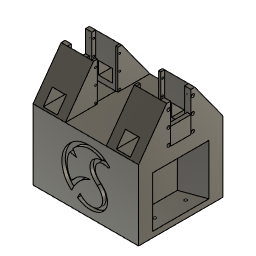
dual_motor_plate v1 (Autodesk Fusion 360 design; units mm, degrees)
Autodesk Fusion 360 part; units mm, degrees
sketch "스케치2" plane through (0, 0, 0) normal (0, 0, 1) x (1, 0, 0)
  line L0 (0, 0) -> (150, 0)
  line L1 (150, 0) -> (150, 120)
  line L2 (150, 120) -> (0, 120)
  line L3 (0, 120) -> (0, 0)
  circle A0 centre (15, 82) radius 2
  circle A1 centre (15, 38) radius 2
  circle A2 centre (135, 82) radius 2
  circle A3 centre (135, 38) radius 2
  line L4 (0, 120) -> (0, 100) construction
  line L5 (0, 0) -> (0, 20) construction
  line L6 (0, 100) -> (35, 100) construction
  line L7 (0, 20) -> (35, 20) construction
  line L8 (32.8892, 88.0293) -> (32.8892, 31.9707) construction
  line L9 (150, 120) -> (150, 100) construction
  line L10 (150, 120) -> (150, 100) construction
  line L11 (32.8892, 88.0293) -> (32.8892, 31.9707)
  line L12 (117.1108, 88.0293) -> (117.1108, 31.9707)
  line L13 (32.8892, 88.0293) -> (0, 100)
  line L14 (32.8892, 31.9707) -> (0, 20)
  line L15 (117.1108, 88.0293) -> (150, 100)
  line L16 (117.1108, 31.9707) -> (150, 20)
  dimension "d15" = 150
  dimension "d16" = 120
  dimension "d19" = 120
  dimension "d20" = 44
  dimension "d21" = 4
  dimension "d22" = 4
  dimension "d23" = 4
  dimension "d24" = 4
  dimension "d98" = 20
  dimension "d99" = 20
  dimension "d100" = 35
  dimension "d102" = 35
  dimension "d105" = 35
  constraint horizontal L0
  constraint vertical L1
  constraint horizontal L2
  constraint vertical L3
  constraint coincident L0.start L3.end
  constraint perpendicular L2 L4
  constraint perpendicular L0 L5
  constraint horizontal L6
  constraint horizontal L7
  constraint coincident L1 L9.end
  constraint parallel L14 L15
  constraint coincident L1 L16.end
  constraint parallel L13 L16
  measures "d15" distance of L0.start L0.end
  measures "d16" distance of L0.start L2.end
  measures "d19" distance of A0.centre A2.centre
  measures "d20" distance of A2.centre A3.centre
  measures "d21" diameter of A0
  measures "d22" diameter of A1
  measures "d23" diameter of A2
  measures "d24" diameter of A3
  measures "d98" distance of L2.end L4.end
  measures "d99" distance of L0.start L5.end
  measures "d100" distance of L4.end L8.start
  measures "d102" distance of L5.end L8.end
  measures "d105" distance of L9.end L12.start
sketch "스케치3" plane through (0, 0, 100) normal (0, 0, 1) x (-1, 0, 0)
  circle A0 centre (-135, -82) radius 2
  circle A1 centre (-15, -82) radius 2
  circle A2 centre (-15, -38) radius 2
  circle A3 centre (-135, -38) radius 2
  line L0 (0, -120) -> (0, 0)
  line L1 (0, 0) -> (-150, 0)
  line L2 (-150, 0) -> (-150, -120)
  line L3 (-150, -120) -> (0, -120)
  line L4 (0, -60) -> (-150, -60) construction
  line L5 (0, -60) -> (-5.5, -60) construction
  line L6 (-5.5, -60) -> (-46.5, -60) construction
  line L7 (-46.5, -60) -> (-103.5, -60) construction
  line L8 (-103.5, -60) -> (-144.5, -60) construction
  line L9 (-144.5, -60) -> (-150, -60) construction
  line L10 (-5.5, -60) -> (-26, -60) construction
  line L11 (-26, -60) -> (-9, -60) construction
  line L12 (-9, -60) -> (-43, -60) construction
  line L13 (-144.5, -60) -> (-124, -60) construction
  line L14 (-124, -60) -> (-141, -60) construction
  line L15 (-141, -60) -> (-107, -60) construction
  line L16 (-46.5, -60) -> (-26, -60) construction
  line L17 (-9, -60) -> (-43, -60) construction
  line L18 (-43, -60) -> (-43, -80) construction
  line L19 (-43, -80) -> (-9, -80) construction
  line L20 (-9, -80) -> (-9, -60) construction
  line L21 (-43, -80) -> (-9, -80)
  line L22 (-9, -80) -> (-9, -40)
  line L23 (-9, -40) -> (-43, -40)
  line L24 (-43, -40) -> (-43, -80)
  line L25 (-107, -60) -> (-141, -60) construction
  line L26 (-141, -60) -> (-141, -40) construction
  line L27 (-141, -40) -> (-107, -40)
  line L28 (-107, -40) -> (-107, -60) construction
  line L29 (-107, -40) -> (-141, -40) construction
  line L30 (-141, -40) -> (-141, -80)
  line L31 (-141, -80) -> (-107, -80)
  line L32 (-107, -80) -> (-107, -40)
  dimension "d27" = 5.5
  dimension "d28" = 41
  dimension "d29" = 57
  dimension "d30" = 41
  dimension "d31" = 5.5
  dimension "d34" = 34
  dimension "d37" = 34
  dimension "d38" = 34
  dimension "d39" = 20
  dimension "d40" = 34
  dimension "d41" = 40
  dimension "d42" = 34
  dimension "d43" = 20
  dimension "d44" = 34
  dimension "d45" = 40
  constraint midpoint L0 L4.start
  constraint midpoint L2 L4.end
  constraint perpendicular L0 L5
  constraint perpendicular L0 L6
  constraint parallel L4 L7
  constraint perpendicular L0 L8
  constraint perpendicular L2 L9
  constraint parallel L4 L10
  constraint parallel L10 L11
  constraint parallel L6 L12
  constraint midpoint L8 L13.end
  constraint parallel L8 L14
  constraint parallel L8 L15
  constraint parallel L12 L16
  constraint horizontal L17
  constraint vertical L18
  constraint horizontal L19
  constraint vertical L20
  constraint horizontal L21
  constraint vertical L22
  constraint horizontal L23
  constraint vertical L24
  constraint horizontal L25
  constraint vertical L26
  constraint horizontal L27
  constraint vertical L28
  constraint horizontal L29
  constraint vertical L30
  constraint horizontal L31
  constraint vertical L32
  measures "d27" distance of L4.start L5.end
  measures "d28" distance of L5.end L6.end
  measures "d29" distance of L6.end L7.end
  measures "d30" distance of L7.end L8.end
  measures "d31" distance of L8.end L4.end
  measures "d34" distance of L11.end L12.end
  measures "d37" distance of L14.end L15.end
  measures "d38" distance of L11.end L12.end
  measures "d39" distance of L11.end L19.end
  measures "d40" distance of L18.end L19.end
  measures "d41" distance of L18.end L23.end
  measures "d42" distance of L15.end L14.end
  measures "d43" distance of L15.end L27.end
  measures "d44" distance of L27.end L26.end
  measures "d45" distance of L27.end L31.end
extrude "돌출3" add sketch "스케치2" along normal blind 100 contours L0 L1 L2 L3 L11 L12 L13 L14 L15 L16 | L3 L11 L13 L14 | L1 L12 L15 L16 | A0 | A1 | A2 | A3 makes body 1
extrude "돌출4" cut sketch "스케치3" against normal blind 5.6 contours L27 L30 L31 L32 | L21 L22 L23 L24 bodies 1
sketch "스케치4" plane through (150, 0, 0) normal (1, 0, 0) x (0, 1, 0)
  line L0 (0, 0) -> (120, 0)
  line L1 (120, 0) -> (120, 100)
  line L2 (120, 100) -> (0, 100)
  line L3 (0, 100) -> (0, 0)
  line L4 (40, 100) -> (80, 100)
  line L5 (40, 100) -> (40, 155.5) construction
  line L6 (80, 100) -> (80, 155.5)
  line L7 (40, 100) -> (45.5, 100)
  line L8 (80, 100) -> (74.5, 100)
  line L9 (45.5, 100) -> (40, 100)
  line L10 (40, 100) -> (40, 155.5)
  line L11 (40, 155.5) -> (45.5, 155.5)
  line L12 (45.5, 155.5) -> (45.5, 100)
  line L13 (74.5, 100) -> (80, 100)
  line L14 (80, 100) -> (80, 155.5) construction
  line L15 (80, 155.5) -> (74.5, 155.5)
  line L16 (74.5, 155.5) -> (74.5, 100)
  line L17 (40, 155.5) -> (0, 100)
  line L18 (80, 155.5) -> (120, 100)
  line L19 (42.75, 155.5) -> (42.75, 146.5) construction
  line L20 (42.75, 146.5) -> (42.75, 124.5) construction
  line L21 (42.75, 124.5) -> (42.75, 102.5) construction
  circle A0 centre (42.75, 146.5) radius 1.25
  circle A1 centre (42.75, 124.5) radius 1.25
  circle A2 centre (42.75, 102.5) radius 1.25
  line L22 (77.25, 155.5) -> (77.25, 146.5) construction
  line L23 (77.25, 146.5) -> (77.25, 124.5) construction
  line L24 (77.25, 124.5) -> (77.25, 102.5) construction
  circle A3 centre (77.25, 146.5) radius 1.25
  circle A4 centre (77.25, 124.5) radius 1.25
  circle A5 centre (77.25, 102.5) radius 1.25
  circle A6 centre (42.75, 146.5) radius 2.25
  circle A7 centre (42.75, 124.5) radius 2.25
  circle A8 centre (42.75, 102.5) radius 2.25
  circle A9 centre (77.25, 102.5) radius 2.25
  circle A10 centre (77.25, 124.5) radius 2.25
  circle A11 centre (77.25, 146.5) radius 2.25
  line L25 (45.5, 124.5) -> (74.5, 124.5)
  line L26 (74.5, 124.5) -> (74.5, 100)
  line L27 (74.5, 100) -> (45.5, 100)
  line L28 (45.5, 100) -> (45.5, 124.5)
  dimension "d50" = 55.5
  dimension "d51" = 55.5
  dimension "d52" = 5.5
  dimension "d53" = 5.5
  dimension "d54" = 9
  dimension "d55" = 22
  dimension "d56" = 22
  dimension "d57" = 2.5
  dimension "d58" = 2.5
  dimension "d59" = 2.5
  dimension "d60" = 9
  dimension "d61" = 22
  dimension "d62" = 22
  dimension "d63" = 2.5
  dimension "d64" = 2.5
  dimension "d65" = 2.5
  dimension "d74" = 4.5
  dimension "d75" = 4.5
  dimension "d76" = 4.5
  dimension "d77" = 4.5
  dimension "d78" = 4.5
  dimension "d79" = 4.5
  constraint coincident L2 L4.start
  constraint coincident L2 L4.end
  constraint perpendicular L3 L4
  constraint perpendicular L4 L5
  constraint perpendicular L4 L6
  constraint perpendicular L5 L7
  constraint perpendicular L6 L8
  constraint horizontal L9
  constraint vertical L10
  constraint horizontal L11
  constraint vertical L12
  constraint horizontal L13
  constraint vertical L14
  constraint horizontal L15
  constraint vertical L16
  constraint coincident L2.end L3.start
  constraint coincident L1.end L2.start
  constraint midpoint L11 L19.start
  constraint perpendicular L11 L19
  constraint parallel L10 L20
  constraint parallel L12 L21
  constraint coincident L19.end L20.start
  constraint coincident L20.end L21.start
  constraint coincident L21.end A2.centre
  constraint midpoint L15 L22.start
  constraint perpendicular L15 L22
  constraint parallel L22 L23
  constraint parallel L23 L24
  constraint coincident L22.end L23.start
  constraint coincident L23.end L24.start
  constraint coincident L24.end A5.centre
  constraint concentric A0 A6
  constraint concentric A1 A7
  constraint concentric A2 A8
  constraint concentric A5 A9
  constraint concentric A3 A11
  constraint horizontal L25
  constraint vertical L26
  constraint horizontal L27
  constraint vertical L28
  constraint coincident L12 L25.start
  measures "d50" distance of L4.start L5.end
  measures "d51" distance of L4.end L6.end
  measures "d52" distance of L4.start L7.end
  measures "d53" distance of L4.end L8.end
  measures "d54" distance of L19.start L19.end
  measures "d55" distance of L19.end L20.end
  measures "d56" distance of L20.end L21.end
  measures "d57" diameter of A0
  measures "d58" diameter of A1
  measures "d59" diameter of A2
  measures "d60" distance of L22.start L22.end
  measures "d61" distance of L22.end L23.end
  measures "d62" distance of L23.end L24.end
  measures "d63" diameter of A3
  measures "d64" diameter of A4
  measures "d65" diameter of A5
  measures "d74" diameter of A6
  measures "d75" diameter of A7
  measures "d76" diameter of A8
  measures "d77" diameter of A9
  measures "d78" diameter of A10
  measures "d79" diameter of A11
extrude "돌출5" add sketch "스케치4" along normal blind 3 separate body contours L2 L10 L17 | L2 L6 L18 | L2 L4 L7 L9 L10 L11 L12 L28 | L2 L4 L6 L8 L13 L15 L16 L26 | A6 | A7 | A8 | A9 | A10 | A11 makes body 2 at (150, 27.7492, 109) makes body 3 at (150, 92.2508, 109)
combine "결합1" operation add target body 2 tool bodies 3 makes body 4 at (150, 92.2508, 109)
move_body "이동1" bodies 2 4 to x (1, 0, 0) y (0, 1, 0) z (0, 0, 1) at (-9, 0, 0)
copy_body "CopyPasteBodies1" bodies 2 4 makes body 5 makes body 6
move_body "이동2" bodies 5 6 to x (1, 0, 0) y (0, 1, 0) z (0, 0, 1) at (-37, 0, 0)
copy_body "CopyPasteBodies2" bodies 2 6 5 4 makes body 7 makes body 8 makes body 9 makes body 10
move_body "이동3" bodies 7 8 10 9 to x (1, 0, 0) y (0, 1, 0) z (0, 0, 1) at (-98, 0, 0)
extrude "돌출7" add 1 faces at (144, 27.7492, 109) along direction (1, 0, 0) up to surface (6 mm away) on bodies 2 bodies 2 4 5 6 7 8 9 10 1
extrude "돌출8" add 1 faces at (144, 92.2508, 109) along direction (1, 0, 0) blind 6 on bodies 4 bodies 4 5 6 7 8 9 10 2
extrude "돌출9" cut sketch "스케치4" against normal blind 6 contours A0 | A1 | A2 | A3 | A4 | A5 | A6 | A7 | A8 | A9 | A10 | A11 bodies 4
extrude "돌출10" add sketch "스케치4" along normal blind 6 separate body contours L2 L10 L17 | L2 L6 L18 | L2 L4 L7 L9 L10 L11 L12 L28 | L2 L4 L6 L8 L13 L15 L16 L26 makes body 11 at (150, 27.1485, 109) makes body 12 at (150, 92.8515, 109)
move_body "이동4" bodies 11 12 to x (1, 0, 0) y (0, 1, 0) z (0, 0, 1) at (-150, 0, 0)
combine "결합2" operation add target body 12 tool bodies 8 11 9 makes body 13 at (9, 27.7492, 109)
extrude "돌출11" add sketch "스케치4" against normal blind 43 contours L2 L10 L17 | L2 L6 L18 bodies 4 5 6
extrude "돌출12" add sketch "스케치4" along normal blind 34 separate body contours L2 L10 L17 | L2 L6 L18 makes body 14 at (161.3333, 93.3333, 137) makes body 15 at (161.3333, 26.6667, 137)
move_body "이동5" bodies 15 14 to x (1, 0, 0) y (0, 1, 0) z (0, 0, 1) at (-141, 0, 0)
extrude "돌출13" add sketch "스케치4" against normal blind 5.4 separate body contours L2 L4 L12 L16 L25 L26 L27 L28 makes body 16
copy_body "CopyPasteBodies3" bodies 16 makes body 17
move_body "이동6" bodies 17 to x (1, 0, 0) y (0, 1, 0) z (0, 0, 1) at (-144.6, 0, 0)
sketch "스케치5" plane through (0, 0, 0) normal (0, -1, 0) x (1, 0, 0)
  line L0 (0, 0) -> (150, 0)
  line L1 (150, 0) -> (150, 100)
  line L2 (150, 100) -> (104, 100)
  line L3 (104, 100) -> (0, 100)
  line L4 (0, 100) -> (0, 0)
  line L5 (127, 100) -> (117, 100)
  line L6 (117, 120) -> (137, 120)
  line L7 (137, 120) -> (137, 102)
  line L8 (137, 102) -> (117, 102)
  line L9 (117, 102) -> (117, 120)
  line L10 (13, 102) -> (33, 102)
  line L11 (33, 102) -> (33, 120)
  line L12 (33, 120) -> (13, 120)
  line L13 (13, 120) -> (13, 102)
  dimension "d90" = 20
  dimension "d92" = 20
  dimension "d94" = 20
  dimension "d95" = 18
  constraint midpoint L2 L5.start
  constraint coincident L2 L5.end
  constraint perpendicular L1 L5
  constraint horizontal L6
  constraint vertical L7
  constraint horizontal L8
  constraint vertical L9
  constraint horizontal L10
  constraint vertical L11
  constraint horizontal L12
  constraint vertical L13
  measures "d90" distance of L5.end L6.start
  measures "d92" distance of L6.start L6.end
  measures "d94" distance of L10.start L10.end
  measures "d95" distance of L10.start L12.end
combine "결합3" operation add target body 15 tool bodies 14 13 12 10 7 4
extrude "돌출14" cut sketch "스케치5" against normal blind 120 contours L6 L7 L8 L9 | L10 L11 L12 L13 bodies 15
sketch "스케치6" plane through (0, 120, 0) normal (0, 1, 0) x (-1, 0, 0)
  line L0 (-150, 0) -> (0, 0)
  line L1 (0, 0) -> (0, 100)
  line L2 (0, 100) -> (-46, 100)
  line L3 (-46, 100) -> (-104, 100)
  line L4 (-104, 100) -> (-150, 100)
  line L5 (-150, 100) -> (-150, 0)
  line L6 (-110, 84) -> (-40, 84)
  line L7 (-40, 84) -> (-40, 16)
  line L8 (-40, 16) -> (-110, 16)
  line L9 (-110, 16) -> (-110, 84)
  line L10 (-75, 80.8) -> (-102.5, 80.8) construction
  line L11 (-102.5, 80.8) -> (-47.5, 80.8) construction
  line L12 (-47.5, 80.8) -> (-47.5, 19.2) construction
  line L13 (-47.5, 19.2) -> (-102.5, 19.2) construction
  line L14 (-102.5, 19.2) -> (-102.5, 80.8) construction
  circle A0 centre (-102.5, 80.8) radius 1.5
  circle A1 centre (-47.5, 80.8) radius 1.5
  circle A2 centre (-102.5, 19.2) radius 1.5
  circle A3 centre (-47.5, 19.2) radius 1.5
  dimension "d110" = 70
  dimension "d111" = 68
  dimension "d116" = 55
  dimension "d117" = 61.6
  dimension "d118" = 3
  dimension "d119" = 3
  dimension "d120" = 3
  dimension "d121" = 3
  constraint horizontal L6
  constraint vertical L7
  constraint horizontal L8
  constraint vertical L9
  constraint horizontal L11
  constraint vertical L12
  constraint horizontal L13
  constraint vertical L14
  constraint coincident L10.end L11.start
  constraint coincident L11.end L12.start
  constraint coincident L13.end L14.start
  constraint coincident L12.end L13.start
  measures "d110" distance of L6.start L6.end
  measures "d111" distance of L6.start L8.end
  measures "d116" distance of L10.end L11.end
  measures "d117" distance of L10.end L13.end
  measures "d118" diameter of A0
  measures "d119" diameter of A1
  measures "d120" diameter of A2
  measures "d121" diameter of A3
extrude "돌출15" cut sketch "스케치6" against normal blind 5 contours L6 L7 L8 L9 | A0 | A1 | A2 | A3 bodies 15
extrude "돌출16" cut sketch "스케치6" against normal blind 10 contours A0 | A1 | A2 | A3 bodies 15
extrude "돌출17" cut sketch "스케치2" along normal blind 80 contours L3 L11 L13 L14 | L1 L12 L15 L16 | A0 | A1 | A2 | A3 bodies 15
extrude "돌출18" add sketch "스케치2" along normal blind 8 contours L3 L11 L13 L14 | L1 L12 L15 L16 bodies 15
sketch "스케치7" plane through (0, 0, 0) normal (0, -1, 0) x (1, 0, 0)
  line L0 (0, 0) -> (150, 0)
  line L1 (150, 0) -> (150, 100)
  line L2 (150, 100) -> (104, 100)
  line L3 (104, 100) -> (46, 100)
  line L4 (46, 100) -> (0, 100)
  line L5 (0, 100) -> (0, 0)
sketch "스케치8" plane through (75, 0, 50) normal (0, -1, 0) x (1, 0, 0)
  spline S0 degree 5 poles (-20.1512, -28.9535) (-20.3666, -28.7887) (-20.8036, -28.4443) (-21.4782, -27.8837) (-22.4158, -27.0479) (-23.6508, -25.8441) (-24.9472, -24.4441) (-26.2998, -22.7858) (-27.6927, -20.8074) (-29.0947, -18.466) (-30.4521, -15.7602) (-31.6969, -12.7202) (-32.755, -9.398) (-33.5542, -5.8575) (-34.0317, -2.165) (-34.1436, 1.621) (-33.8627, 5.4488) (-33.1759, 9.2713) (-32.0819, 13.0444) (-30.5889, 16.7249) (-28.7125, 20.2689) (-26.474, 23.6297) (-23.8981, 26.7595) (-21.0116, 29.6118) (-17.8418, 32.143) (-14.4143, 34.3146) (-10.7522, 36.0953) (-6.8741, 37.4635) (-2.7941, 38.4064) (1.4776, 38.9177) (5.9341, 38.9955) (9.6436, 38.7117) (12.5061, 38.305) (14.4501, 37.9479) (15.4309, 37.7479) knots 0 0 0 0 0 0 0.033333 0.066667 0.1 0.133333 0.166667 0.2 0.233333 0.266667 0.3 0.333333 0.366667 0.4 0.433333 0.466667 0.5 0.533333 0.566667 0.6 0.633333 0.666667 0.7 0.733333 0.766667 0.8 0.833333 0.866667 0.9 0.933333 0.966667 1 1 1 1 1 1
  spline S1 degree 5 poles (15.4309, 37.7479) (15.6205, 37.7339) (16.0093, 37.6921) (16.6216, 37.5882) (17.4968, 37.3668) (18.6893, 36.9498) (19.977, 36.3929) (21.3504, 35.7016) (22.7884, 34.8915) (24.2597, 33.9875) (25.7275, 33.0192) (27.1535, 32.018) (28.502, 31.0132) (29.7439, 30.0294) (30.8625, 29.0822) (31.8507, 28.1797) (32.5363, 27.496) (32.9922, 27.0049) (33.2703, 26.687) (33.4029, 26.5305) knots 0 0 0 0 0 0 0.066667 0.133333 0.2 0.266667 0.333333 0.4 0.466667 0.533333 0.6 0.666667 0.733333 0.8 0.866667 0.933333 1 1 1 1 1 1
  spline S2 degree 5 poles (33.4029, 26.5305) (33.4205, 26.4745) (33.4487, 26.3561) (33.4707, 26.1597) (33.4592, 25.8606) (33.3718, 25.4401) (33.1937, 25.0294) (32.8993, 24.714) (32.4701, 24.5642) (31.9107, 24.5893) (31.2465, 24.7436) (30.5109, 24.9601) (29.7369, 25.1747) (28.9454, 25.3561) (28.1471, 25.498) (27.3449, 25.608) (26.5357, 25.6985) (25.7123, 25.7757) (24.866, 25.8322) (23.9882, 25.8516) (23.0728, 25.8122) (22.118, 25.6905) (21.1289, 25.4655) (20.119, 25.1217) (19.108, 24.6488) (18.1191, 24.0417) (17.1775, 23.3004) (16.3073, 22.4291) (15.5299, 21.4368) (14.8611, 20.337) (14.3118, 19.1464) (13.8885, 17.8841) (13.5945, 16.5704) (13.4306, 15.2255) (13.3959, 13.8686) (13.4882, 12.5166) (13.7055, 11.1831) (14.046, 9.8779) (14.5079, 8.608) (15.0898, 7.3779) (15.7905, 6.1901) (16.4455, 5.2747) (16.9895, 4.6078) (17.3757, 4.172) (17.5747, 3.9563) knots 0 0 0 0 0 0 0.025 0.05 0.075 0.1 0.125 0.15 0.175 0.2 0.225 0.25 0.275 0.3 0.325 0.35 0.375 0.4 0.425 0.45 0.475 0.5 0.525 0.55 0.575 0.6 0.625 0.65 0.675 0.7 0.725 0.75 0.775 0.8 0.825 0.85 0.875 0.9 0.925 0.95 0.975 1 1 1 1 1 1
  spline S3 degree 5 poles (17.5747, 3.9563) (17.6741, 3.8277) (17.8885, 3.5636) (18.2573, 3.1465) (18.8433, 2.5486) (19.7281, 1.7294) (20.7502, 0.8335) (21.8784, -0.1497) (23.0699, -1.2323) (24.2769, -2.4237) (25.4522, -3.7271) (26.5556, -5.1338) (27.5578, -6.6232) (28.4379, -8.1696) (29.1833, -9.7476) (29.788, -11.3375) (30.2521, -12.9326) (30.58, -14.54) (30.7767, -16.1736) (30.8449, -17.8481) (30.7817, -19.5736) (30.5749, -21.3484) (30.2051, -23.1596) (29.6508, -24.9867) (28.8931, -26.8039) (27.92, -28.5832) (26.7315, -30.2974) (25.3412, -31.9215) (23.7711, -33.433) (22.0488, -34.8119) (20.2036, -36.0406) (18.2635, -37.105) (16.2506, -37.9935) (14.1805, -38.6983) (12.0651, -39.2153) (9.9145, -39.5441) (7.7396, -39.689) (5.554, -39.6589) (3.3762, -39.4679) (1.2312, -39.1351) (-0.8537, -38.682) (-2.8501, -38.131) (-4.7313, -37.5035) (-6.4747, -36.8178) (-8.0644, -36.087) (-9.4914, -35.319) (-10.4995, -34.678) (-11.1799, -34.1828) (-11.6, -33.8464) (-11.8016, -33.6766) knots 0 0 0 0 0 0 0.022222 0.044444 0.066667 0.088889 0.111111 0.133333 0.155556 0.177778 0.2 0.222222 0.244444 0.266667 0.288889 0.311111 0.333333 0.355556 0.377778 0.4 0.422222 0.444444 0.466667 0.488889 0.511111 0.533333 0.555556 0.577778 0.6 0.622222 0.644444 0.666667 0.688889 0.711111 0.733333 0.755556 0.777778 0.8 0.822222 0.844444 0.866667 0.888889 0.911111 0.933333 0.955556 0.977778 1 1 1 1 1 1
  line L0 (-11.8016, -33.6766) -> (-8.1599, -26.9758)
  spline S4 degree 5 poles (-8.1599, -26.9758) (-8.0677, -27.0973) (-7.8739, -27.3434) (-7.5554, -27.722) (-7.0748, -28.246) (-6.3818, -28.9313) (-5.5992, -29.6427) (-4.734, -30.3707) (-3.7948, -31.1018) (-2.7893, -31.8188) (-1.7215, -32.5026) (-0.5877, -33.1329) (0.6216, -33.6896) (1.9161, -34.1547) (3.3001, -34.5144) (4.7673, -34.7606) (6.2945, -34.893) (7.8461, -34.9174) (9.3824, -34.8426) (10.8664, -34.6771) (12.2709, -34.4266) (13.5873, -34.0905) (14.8248, -33.6618) (16.0009, -33.1299) (17.134, -32.4828) (18.2361, -31.7094) (19.3035, -30.8019) (20.3208, -29.7565) (21.2642, -28.5734) (22.1063, -27.2572) (22.8195, -25.8173) (23.3806, -24.2686) (23.7709, -22.6299) (23.9755, -20.9221) (23.9832, -19.1666) (23.7853, -17.3837) (23.376, -15.5908) (22.7516, -13.8008) (21.9099, -12.023) (20.8503, -10.2633) (19.5728, -8.5252) (18.377, -7.1534) (17.3826, -6.1353) (16.6763, -5.4614) (16.3124, -5.1256) knots 0 0 0 0 0 0 0.025 0.05 0.075 0.1 0.125 0.15 0.175 0.2 0.225 0.25 0.275 0.3 0.325 0.35 0.375 0.4 0.425 0.45 0.475 0.5 0.525 0.55 0.575 0.6 0.625 0.65 0.675 0.7 0.725 0.75 0.775 0.8 0.825 0.85 0.875 0.9 0.925 0.95 0.975 1 1 1 1 1 1
  spline S5 degree 5 poles (16.3124, -5.1256) (16.147, -4.988) (15.8142, -4.7057) (15.3085, -4.2605) (14.6212, -3.6235) (13.7414, -2.755) (12.845, -1.8155) (11.9396, -0.8076) (11.0387, 0.2637) (10.1608, 1.3912) (9.3268, 2.5672) (8.5577, 3.7842) (7.8719, 5.0362) (7.2828, 6.3204) (6.7974, 7.6369) (6.4186, 8.9868) (6.1465, 10.3699) (5.9808, 11.7828) (5.9219, 13.217) (5.9726, 14.6569) (6.1365, 16.0837) (6.4174, 17.4772) (6.818, 18.8192) (7.3389, 20.0954) (7.9776, 21.2988) (8.7291, 22.4268) (9.5861, 23.4796) (10.5399, 24.4578) (11.5799, 25.3608) (12.6951, 26.1847) (13.8739, 26.9235) (15.1056, 27.5705) (16.3802, 28.1188) (17.69, 28.563) (19.0298, 28.8998) (20.3962, 29.1277) (21.5094, 29.2224) (22.3552, 29.2444) (22.9239, 29.2372) (23.2095, 29.2281) knots 0 0 0 0 0 0 0.028571 0.057143 0.085714 0.114286 0.142857 0.171429 0.2 0.228571 0.257143 0.285714 0.314286 0.342857 0.371429 0.4 0.428571 0.457143 0.485714 0.514286 0.542857 0.571429 0.6 0.628571 0.657143 0.685714 0.714286 0.742857 0.771429 0.8 0.828571 0.857143 0.885714 0.914286 0.942857 0.971429 1 1 1 1 1 1
  spline S6 degree 5 poles (23.2095, 29.2281) (23.1228, 29.3204) (22.934, 29.5059) (22.6042, 29.7871) (22.0713, 30.1676) (21.2528, 30.6514) (20.292, 31.1391) (19.2109, 31.6224) (18.0391, 32.0901) (16.8085, 32.5316) (15.5489, 32.9383) (14.2816, 33.307) (13.0184, 33.6389) (11.7617, 33.9358) (10.5047, 34.1974) (9.2313, 34.4181) (7.9163, 34.5845) (6.5307, 34.6781) (5.048, 34.6792) (3.4492, 34.5695) (1.7287, 34.3358) (-0.1008, 33.9727) (-2.0137, 33.4806) (-3.9751, 32.8642) (-5.9455, 32.1314) (-7.8849, 31.2913) (-9.7564, 30.3533) (-11.5315, 29.3253) (-13.191, 28.2133) (-14.7227, 27.0216) (-16.1201, 25.7531) (-17.1283, 24.6784) (-17.8226, 23.839) (-18.2581, 23.2646) (-18.4689, 22.9737) knots 0 0 0 0 0 0 0.033333 0.066667 0.1 0.133333 0.166667 0.2 0.233333 0.266667 0.3 0.333333 0.366667 0.4 0.433333 0.466667 0.5 0.533333 0.566667 0.6 0.633333 0.666667 0.7 0.733333 0.766667 0.8 0.833333 0.866667 0.9 0.933333 0.966667 1 1 1 1 1 1
  line L1 (-18.4689, 22.9737) -> (-13.116, 14.972)
  line L2 (-13.116, 14.972) -> (-22.6077, 17.0138)
  spline S7 degree 5 poles (-22.6077, 17.0138) (-22.6914, 16.8989) (-22.8587, 16.6563) (-23.1088, 16.2536) (-23.4411, 15.6391) (-23.8536, 14.743) (-24.2614, 13.7245) (-24.6606, 12.5974) (-25.0454, 11.3828) (-25.4082, 10.1038) (-25.741, 8.7819) (-26.035, 7.433) (-26.2814, 6.0627) (-26.4719, 4.669) (-26.5985, 3.2462) (-26.654, 1.7874) (-26.6321, 0.2878) (-26.5281, -1.2516) (-26.3381, -2.8254) (-26.0596, -4.425) (-25.6907, -6.0406) (-25.2307, -7.6623) (-24.6794, -9.2816) (-24.0376, -10.8928) (-23.3063, -12.4922) (-22.4868, -14.0778) (-21.7615, -15.3344) (-21.1787, -16.2701) (-20.7731, -16.8909) (-20.5659, -17.2005) knots 0 0 0 0 0 0 0.04 0.08 0.12 0.16 0.2 0.24 0.28 0.32 0.36 0.4 0.44 0.48 0.52 0.56 0.6 0.64 0.68 0.72 0.76 0.8 0.84 0.88 0.92 0.96 1 1 1 1 1 1
  spline S8 degree 5 poles (-20.5659, -17.2005) (-20.5426, -17.162) (-20.483, -17.0727) (-20.3543, -16.9024) (-20.1043, -16.6023) (-19.664, -16.1076) (-19.1088, -15.5029) (-18.4609, -14.8057) (-17.7447, -14.0369) (-16.9804, -13.219) (-16.1775, -12.3714) (-15.3298, -11.5085) (-14.4217, -10.6412) (-13.4332, -9.7779) (-12.3459, -8.926) (-11.1474, -8.0927) (-9.8382, -7.2867) (-8.432, -6.5182) (-6.951, -5.7981) (-5.4229, -5.1375) (-3.8782, -4.5468) (-2.3462, -4.0355) (-0.8526, -3.6108) (0.5846, -3.2775) (1.9541, -3.0379) (3.2497, -2.8927) (4.2249, -2.8519) (4.9216, -2.8635) (5.3708, -2.8899) (5.5915, -2.9078) knots 0 0 0 0 0 0 0.04 0.08 0.12 0.16 0.2 0.24 0.28 0.32 0.36 0.4 0.44 0.48 0.52 0.56 0.6 0.64 0.68 0.72 0.76 0.8 0.84 0.88 0.92 0.96 1 1 1 1 1 1
  spline S9 degree 5 poles (5.5915, -2.9078) (5.4632, -2.9702) (5.2025, -3.0965) (4.7993, -3.2902) (4.2372, -3.5569) (3.4922, -3.9061) (2.7001, -4.2756) (1.8522, -4.6744) (0.9379, -5.1152) (-0.052, -5.6133) (-1.122, -6.1854) (-2.2695, -6.8484) (-3.4862, -7.618) (-4.76, -8.5065) (-6.0754, -9.5218) (-7.4154, -10.6645) (-8.7627, -11.927) (-10.0997, -13.2951) (-11.4098, -14.7504) (-12.6773, -16.2722) (-13.8883, -17.8396) (-15.0314, -19.4332) (-16.098, -21.0375) (-17.083, -22.6418) (-17.9836, -24.2389) (-18.7986, -25.8249) (-19.3822, -27.0832) (-19.7815, -28.0208) (-20.0308, -28.6431) (-20.1512, -28.9535) knots 0 0 0 0 0 0 0.04 0.08 0.12 0.16 0.2 0.24 0.28 0.32 0.36 0.4 0.44 0.48 0.52 0.56 0.6 0.64 0.68 0.72 0.76 0.8 0.84 0.88 0.92 0.96 1 1 1 1 1 1
  point P0 (-23.1666, -26.3)
  point P1 (-27.7501, -20.6309)
  point P2 (-33.5397, -5.4331)
  point P3 (-30.4037, 16.8811)
  point P4 (-13.3966, 34.7325)
  point P5 (20.6175, 36.0593)
  point P6 (28.8195, 30.7521)
  point P7 (33.4029, 25.6379)
  point P8 (32.7436, 24.6899)
  point P9 (30.4352, 24.9784)
  point P10 (26.6842, 25.6791)
  point P11 (22.1913, 25.6791)
  point P12 (16.1732, 22.2167)
  point P13 (13.4527, 13.272)
  point P14 (19.8883, 1.5968)
  point P15 (24.9908, -3.238)
  point P16 (29.5222, -10.6872)
  point P17 (30.8063, -18.3814)
  point P18 (28.33, -27.777)
  point P19 (19.1529, -36.5899)
  point P20 (6.4069, -39.6489)
  point P21 (-5.5379, -37.1726)
  point P22 (-6.1205, -29.1608)
  point P23 (-2.2603, -32.147)
  point P24 (3.6392, -34.5506)
  point P25 (11.5053, -34.5506)
  point P26 (17.2592, -32.3655)
  point P27 (22.2119, -26.9758)
  point P28 (23.7414, -17.4346)
  point P29 (12.3866, -1.2972)
  point P30 (8.1085, 4.6328)
  point P31 (6.033, 11.4946)
  point P32 (6.8273, 18.7435)
  point P33 (10.4678, 24.3499)
  point P34 (16.3124, 28.0631)
  point P35 (21.1238, 30.703)
  point P36 (16.3124, 32.6862)
  point P37 (10.5581, 34.1761)
  point P38 (3.66, 34.5624)
  point P39 (-8.8116, 30.8099)
  point P40 (-24.0425, 14.2546)
  point P41 (-25.7532, 8.6809)
  point P42 (-26.6362, 1.5622)
  point P43 (-25.3118, -7.3225)
  point P44 (-19.8485, -16.3176)
  point P45 (-17.0893, -13.3376)
  point P46 (-11.8468, -8.5918)
  point P47 (-2.024, -3.9563)
  point P48 (3.3841, -3.9563)
  point P49 (0.0731, -5.5566)
  point P50 (-6.0524, -9.5299)
  point P51 (-14.606, -18.8561)
extrude "돌출19" cut sketch "스케치8" against normal blind 5 bodies 15
thread "스레드1" "ISO Metric profile 4.5 M4.5x0.75 6H" major diameter 4.6131 minor diameter 3.7831 pitch 0.75 angle 60 resizes the face on face at (136.3234, 83.4996, 5.3333) on bodies 15
thread "스레드2" "ISO Metric profile 4.5 M4.5x0.75 6H" major diameter 4.6131 minor diameter 3.7831 pitch 0.75 angle 60 resizes the face on face at (136.0851, 39.6801, 5.3333) on bodies 15
thread "스레드3" "ISO Metric profile 4.5 M4.5x0.75 6H" major diameter 4.6131 minor diameter 3.7831 pitch 0.75 angle 60 resizes the face on face at (16.9975, 37.9003, 5.3333) on bodies 15
thread "스레드4" "ISO Metric profile 4.5 M4.5x0.75 6H" major diameter 4.6131 minor diameter 3.7831 pitch 0.75 angle 60 resizes the face on face at (16.843, 82.7769, 5.3333) on bodies 15
thread "스레드5" "ISO Metric profile 3.5 M3.5x0.6 6H" major diameter 3.5995 minor diameter 2.93 pitch 0.6 angle 60 resizes the face on face at (101.3043, 111.6667, 81.7057) on bodies 15
thread "스레드6" "ISO Metric profile 3.5 M3.5x0.6 6H" major diameter 3.5995 minor diameter 2.93 pitch 0.6 angle 60 resizes the face on face at (46.0905, 111.6667, 81.313) on bodies 15
thread "스레드7" "ISO Metric profile 3.5 M3.5x0.6 6H" major diameter 3.5995 minor diameter 2.93 pitch 0.6 angle 60 resizes the face on face at (101.3043, 111.6667, 20.1057) on bodies 15
thread "스레드8" "ISO Metric profile 3.5 M3.5x0.6 6H" major diameter 3.5995 minor diameter 2.93 pitch 0.6 angle 60 resizes the face on face at (48.4925, 111.6667, 18.0753) on bodies 15
thread "스레드9" "ISO Metric profile 3.0 M3x0.5 6H" major diameter 3.086 minor diameter 2.529 pitch 0.5 angle 60 resizes the face on face at (143, 43.5771, 147.4372) on bodies 15
thread "스레드10" "ISO Metric profile 3.0 M3x0.5 6H" major diameter 3.086 minor diameter 2.529 pitch 0.5 angle 60 resizes the face on face at (143, 43.9613, 124.8084) on bodies 15
thread "스레드11" "ISO Metric profile 3.0 M3x0.5 6H" major diameter 3.086 minor diameter 2.529 pitch 0.5 angle 60 resizes the face on face at (143, 43.9613, 102.8084) on bodies 15
thread "스레드12" "ISO Metric profile 3.0 M3x0.5 6H" major diameter 3.086 minor diameter 2.529 pitch 0.5 angle 60 resizes the face on face at (142, 77.6481, 147.6849) on bodies 15
thread "스레드13" "ISO Metric profile 3.0 M3x0.5 6H" major diameter 3.086 minor diameter 2.529 pitch 0.5 angle 60 resizes the face on face at (142, 77.6481, 125.6849) on bodies 15
thread "스레드14" "ISO Metric profile 3.0 M3x0.5 6H" major diameter 3.086 minor diameter 2.529 pitch 0.5 angle 60 resizes the face on face at (142, 76.0106, 124.2494) on bodies 15
thread "스레드15" "ISO Metric profile 3.0 M3x0.5 6H" major diameter 3.086 minor diameter 2.529 pitch 0.5 angle 60 resizes the face on face at (142, 77.6481, 103.6849) on bodies 15
thread "스레드16" "ISO Metric profile 3.0 M3x0.5 6H" major diameter 3.086 minor diameter 2.529 pitch 0.5 angle 60 resizes the face on face at (8, 77.5886, 147.7033) on bodies 15
thread "스레드17" "ISO Metric profile 3.0 M3x0.5 6H" major diameter 3.086 minor diameter 2.529 pitch 0.5 angle 60 resizes the face on face at (8, 41.9229, 145.5628) on bodies 15
thread "스레드18" "ISO Metric profile 3.0 M3x0.5 6H" major diameter 3.086 minor diameter 2.529 pitch 0.5 angle 60 resizes the face on face at (8, 77.5886, 125.7033) on bodies 15
thread "스레드19" "ISO Metric profile 3.0 M3x0.5 6H" major diameter 3.086 minor diameter 2.529 pitch 0.5 angle 60 resizes the face on face at (8, 43.9613, 124.8084) on bodies 15
thread "스레드20" "ISO Metric profile 3.0 M3x0.5 6H" major diameter 3.086 minor diameter 2.529 pitch 0.5 angle 60 resizes the face on face at (8, 77.5886, 103.7033) on bodies 15
thread "스레드21" "ISO Metric profile 3.0 M3x0.5 6H" major diameter 3.086 minor diameter 2.529 pitch 0.5 angle 60 resizes the face on face at (8, 43.9613, 102.8084) on bodies 15
thread "스레드22" "ISO Metric profile 3.0 M3x0.5 6H" major diameter 3.086 minor diameter 2.529 pitch 0.5 angle 60 resizes the face on face at (45, 41.9229, 145.5628) on bodies 15
thread "스레드23" "ISO Metric profile 3.0 M3x0.5 6H" major diameter 3.086 minor diameter 2.529 pitch 0.5 angle 60 resizes the face on face at (45, 43.9613, 124.8084) on bodies 15
thread "스레드24" "ISO Metric profile 3.0 M3x0.5 6H" major diameter 3.086 minor diameter 2.529 pitch 0.5 angle 60 resizes the face on face at (45, 43.9613, 102.8084) on bodies 15
thread "스레드25" "ISO Metric profile 3.0 M3x0.5 6H" major diameter 3.086 minor diameter 2.529 pitch 0.5 angle 60 resizes the face on face at (45, 77.5886, 147.7033) on bodies 15
thread "스레드26" "ISO Metric profile 3.0 M3x0.5 6H" major diameter 3.086 minor diameter 2.529 pitch 0.5 angle 60 resizes the face on face at (45, 77.5886, 125.7033) on bodies 15
thread "스레드27" "ISO Metric profile 3.0 M3x0.5 6H" major diameter 3.086 minor diameter 2.529 pitch 0.5 angle 60 resizes the face on face at (45, 77.5886, 103.7033) on bodies 15
thread "스레드28" "ISO Metric profile 3.0 M3x0.5 6H" major diameter 3.086 minor diameter 2.529 pitch 0.5 angle 60 resizes the face on face at (106, 41.9229, 145.5628) on bodies 15
thread "스레드29" "ISO Metric profile 3.0 M3x0.5 6H" major diameter 3.086 minor diameter 2.529 pitch 0.5 angle 60 resizes the face on face at (106, 43.9613, 124.8084) on bodies 15
thread "스레드30" "ISO Metric profile 3.0 M3x0.5 6H" major diameter 3.086 minor diameter 2.529 pitch 0.5 angle 60 resizes the face on face at (106, 43.9613, 102.8084) on bodies 15
thread "스레드31" "ISO Metric profile 3.0 M3x0.5 6H" major diameter 3.086 minor diameter 2.529 pitch 0.5 angle 60 resizes the face on face at (106, 77.5886, 147.7033) on bodies 15
thread "스레드32" "ISO Metric profile 3.0 M3x0.5 6H" major diameter 3.086 minor diameter 2.529 pitch 0.5 angle 60 resizes the face on face at (106, 77.5886, 125.7033) on bodies 15
thread "스레드33" "ISO Metric profile 3.0 M3x0.5 6H" major diameter 3.086 minor diameter 2.529 pitch 0.5 angle 60 resizes the face on face at (106, 77.5886, 103.7033) on bodies 15
